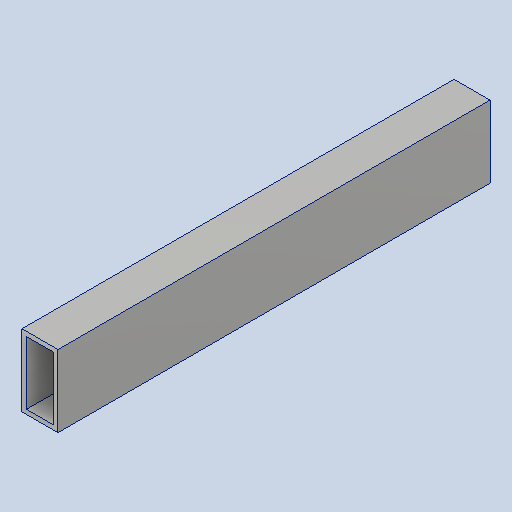
# Autodesk Inventor part: EL1-001
Saved by Autodesk Inventor 2023.4 (Build 274418000, 418)
## iProperties
RuleStatus: InUse
Created: 2025-01-09
Part Number: EL1-001
Material: Aluminum 6061
Document SubType Name: Modeling
Designer: mavericks
Mass: 304.185 g
Surface Area: 718.547 cm^2
Volume: 112.661 cm^3
Density: 2.7 g/cm^3
Appearance: Aluminum - Flat
AfterDocNew0: SHOW
AfterDocOpen0: SHOW
Author: mavericks
Autodesk Inventor part; units mm, degrees
ref_plane "YZ Plane" through (0, 0, 0) normal (1, 0, 0) x (0, 1, 0)
ref_plane "XZ Plane" through (0, 0, 0) normal (0, 1, 0) x (-1, 0, 0)
ref_plane "XY Plane" through (0, 0, 0) normal (0, 0, 1) x (1, 0, 0)
sketch "Sketch1" plane through (0, 0, 0) normal (0, 0, 1) x (1, 0, 0)
  line L0 (-12.7, -25.4) -> (12.7, -25.4)
  line L1 (12.7, -25.4) -> (12.7, 25.4)
  line L2 (12.7, 25.4) -> (-12.7, 25.4)
  line L3 (-12.7, 25.4) -> (-12.7, -25.4)
  line L4 (-12.7, -25.4) -> (12.7, 25.4) construction
  line L5 (12.7, -25.4) -> (-12.7, 25.4) construction
  line L6 (-9.525, 22.225) -> (9.525, 22.225)
  line L7 (9.525, 22.225) -> (9.525, -22.225)
  line L8 (9.525, -22.225) -> (-9.525, -22.225)
  line L9 (-9.525, -22.225) -> (-9.525, 22.225)
  point P0 (0, 0)
  dimension "width" = 25.4
  dimension "height" = 50.8
  dimension "thickness" = 3.175
  constraints: 20 end point, 4 parallel, 2 midpoint, 2 perpendicular, 1 horizontal, 3 other
  measures "width" distance of L2.end L1.end
  measures "height" distance of L1.end L0.end
  measures "thickness" distance between parallel lines of L2 L6
extrude "Extrusion1" add sketch "Sketch1" along normal mid plane 304.8
body "Solid1"
